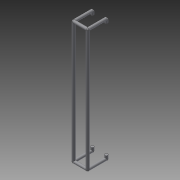
# Autodesk Inventor part: Y_Rail_Bridge-Rod-Rev1
Saved by Autodesk Inventor 2015 (Build 190159000, 159)
## iProperties
Created: 2016-12-21
Part Number: Y_Rail_Bridge-Rod-Rev1
Material: Generic
Document SubType Name: Modeling
Designer: Guy
Density: 1 g/cm^3
Appearance: Default
Author: Guy
Autodesk Inventor part; units mm, degrees
sketch "Sketch1" plane through (0, 0, 0) normal (0, 0, 1) x (1, 0, 0)
  circle A0 centre (0, 0) radius 15
  circle A1 centre (150, 0) radius 15
  line L0 (0, 0) -> (150, 0)
  dimension "d0" = 30
  dimension "d3" = 30
  dimension "d4" = 150
  constraints: 2 centre point, 2 end point, 1 coincident, 1 horizontal
  measures "d0" diameter of A0
  measures "d3" diameter of A1
  measures "d4" distance of L0.end point (0, 0)
extrude "Extrusion1" add sketch "Sketch1" along normal blind 1300
sketch "Sketch2" plane through (0, 0, 0) normal (0, 1, 0) x (-1, 0, 0)
  line L0 (15, 1300) -> (-15, 1300) projected
  line L1 (-15, 0) -> (15, 0) projected
  line L2 (-135, 1300) -> (-165, 1300) projected
  line L3 (-165, 0) -> (-135, 0) projected
  circle A0 centre (0, 0) radius 15
  line L4 (-165, 0) -> (-135, 0) projected
  circle A1 centre (-150, 0) radius 15
  line L5 (15, 1300) -> (-15, 1300) projected
  circle A2 centre (0, 1300) radius 15
  line L6 (-135, 1300) -> (-165, 1300) projected
  circle A3 centre (-150, 1300) radius 15
  constraints: 4 horizontal alignment, 3 midpoint, 1 coincident, 8 other
extrude "Extrusion2" add sketch "Sketch2" along normal blind 200
sketch "Sketch3" plane through (0, 0, 1300) normal (0, 0, 1) x (1, 0, 0)
  line L0 (135, 0) -> (165, 0) projected
  line L1 (165, 0) -> (135, 0) projected
  arc A0 (135, 0) -> (165, 0) centre (150, 0) ccw projected
  line L2 (15, 0) -> (-15, 0) projected
  arc A1 (-15, 0) -> (15, 0) centre (0, 0) ccw projected
  circle A2 centre (150, 0) radius 15
  line L3 (165, 0) -> (135, 0)
  circle A3 centre (0, 0) radius 15
  line L4 (15, 0) -> (-15, 0)
  constraints: 4 end point, 2 centre point, 2 coincident, 2 concentric, 2 horizontal
revolve "Revolution1" add sketch "Sketch3" angle 90 about axis through (135, 0, 1300) along (-1, 0, 0) contours L0 A0 | A1 L2
sketch "Sketch4" plane through (0, 0, 0) normal (0, 0, -1) x (-1, 0, 0)
  line L0 (15, 0) -> (-15, 0) projected
  arc A0 (-15, 0) -> (15, 0) centre (0, 0) ccw projected
  line L1 (-135, 0) -> (-165, 0) projected
  arc A1 (-165, 0) -> (-135, 0) centre (-150, 0) ccw projected
  circle A2 centre (0, 0) radius 15
  circle A3 centre (-150, 0) radius 15
  line L2 (-165, 0) -> (-135, 0)
  line L3 (15, 0) -> (-15, 0)
  constraints: 4 end point, 2 centre point, 2 coincident, 2 horizontal
revolve "Revolution2" add sketch "Sketch4" angle 90 about axis through (-15, 0, 0) along (1, 0, 0) contours A0 L0 | A1 L1
sketch "Sketch5" plane through (150, 200, 1300) normal (0, 1, 0) x (1, 0, 0)
  circle A0 centre (0, 0) radius 15 projected
  circle A1 centre (0, 0) radius 15
  line L0 (-15, 0) -> (0, 0)
  line L1 (0, 0) -> (0, -15)
  point P0 (-150, 1300)
  point P1 (15, 0)
  constraints: 4 end point, 3 point on circle, 1 centre point, 1 coincident, 1 horizontal, 1 perpendicular
extrude "Extrusion4" add sketch "Sketch5" along normal blind 0.01 contours L0 L1 A0 picked at (-1.1126, -9.8746)
ref_plane "Work Plane1" through (150, 200.01, 1300) normal (0, 0, -1) x (-1, 0, 0)
sketch "Sketch6" plane through (150, 200.01, 1300) normal (0, 0, -1) x (-1, 0, 0)
  line L0 (15, -0.01) -> (-15, -0.01) projected
  line L1 (165, -0.01) -> (135, -0.01) projected
  circle A0 centre (150, -0.01) radius 15
  circle A1 centre (0, -0.01) radius 15
  point P0 (150, -200.01)
  constraints: 2 horizontal alignment, 1 coincident, 1 midpoint, 4 other
extrude "Extrusion5" add sketch "Sketch6" along normal blind 1300
ref_plane "Work Plane2" through (150, 200.01, 650) normal (0, 0, 1) x (1, 0, 0)
sketch "Sketch7" plane through (150, 200.01, 650) normal (0, 0, 1) x (1, 0, 0)
  arc A0 (15, -0.01) -> (-15, -0.01) centre (0, -0.01) ccw projected
  arc A1 (-15, -0.01) -> (15, -0.01) centre (0, -0.01) ccw projected
  line L0 (15, -0.01) -> (-15, -0.01) projected
  arc A2 (15, -200.01) -> (-15, -200.01) centre (0, -200.01) ccw projected
  line L1 (-15, -200.01) -> (15, -200.01) projected
  circle A3 centre (0, -0.01) radius 15
  line L2 (-165, -0.01) -> (-135, -0.01) projected
  arc A4 (-135, -0.01) -> (-165, -0.01) centre (-150, -0.01) ccw projected
  arc A5 (-165, -0.01) -> (-135, -0.01) centre (-150, -0.01) ccw projected
  line L3 (-135, -0.01) -> (-165, -0.01) projected
  arc A6 (-135, -200.01) -> (-165, -200.01) centre (-150, -200.01) ccw projected
  line L4 (-165, -200.01) -> (-135, -200.01) projected
  circle A7 centre (-150, -0.01) radius 15
  constraints: 2 coincident, 2 horizontal alignment, 4 other
extrude "Extrusion6" cut sketch "Sketch7" along normal mid plane 1225 contours L0 A0 | A1 L0 | A4 L2 | L2 A5
ref_plane "Work Plane3" through (0, 0, -10) normal (-1, 0, 0) x (0, 0, 1)
sketch "Sketch8" plane through (0, 0, -10) normal (-1, 0, 0) x (0, 0, 1)
  line L0 (1310, 0) -> (1310, 0) projected
  line L1 (1310, 0) -> (1310, 0) projected
  line L2 (10, 0) -> (10, 0) projected
  line L3 (10, 0) -> (10, 0) projected
  line L4 (10, 200) -> (10, 200) projected
  line L5 (10, 200) -> (10, 200) projected
  line L6 (10, 0) -> (10, 0) projected
  line L7 (10, 0) -> (10, 0) projected
  line L8 (25, 15) -> (1295, 15) projected
  line L9 (10, -15) -> (1310, -15) projected
  line L10 (10, 0) -> (10, -15) projected
  line L11 (10, 0) -> (25, 15) projected
  line L12 (25, 15) -> (25, 185) projected
  line L13 (-5, 0) -> (-5, 200) projected
  line L14 (-5, 0) -> (10, 0) projected
  line L15 (1295, 15) -> (1310, 0) projected
  line L16 (1310, 0) -> (1325, 0) projected
  line L17 (1310, -15) -> (1310, 0) projected
  line L18 (1325, 0) -> (1325, 200) projected
  line L19 (1295, 15) -> (1295, 185) projected
  arc A0 (1310, -15) -> (1325, 0) centre (1310, 0) ccw projected
  line L20 (10, 0) -> (10, 0) projected
  line L21 (10, 0) -> (10, 0) projected
  arc A1 (-5, 0) -> (10, -15) centre (10, 0) ccw projected
  circle A2 centre (10, 0) radius 15
  circle A3 centre (1310, 0) radius 15
  constraints: 2 horizontal, 2 vertical, 1 horizontal alignment, 1 vertical alignment, 4 other
extrude "Extrusion7" add sketch "Sketch8" against normal blind 150 contours A2 L10 L11 | L11 L14 A2 | A3 L16 L15 | L15 L17 A3 | L10 A1 L14 | L16 A0 L17
body "Solid1"
